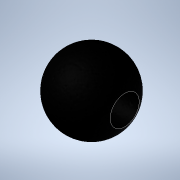
# Autodesk Inventor part: Ball
Saved by Autodesk Inventor 2022 (Build 260153000, 153)
## iProperties
Created: 2023-01-20
Part Number: Ball
Material: Generic
Document SubType Name: Modeling
Designer: ASUS
Density: 1 g/cm^3
Appearance: Fine Textured - Black
Author: ASUS
Autodesk Inventor part; units mm, degrees
ref_plane "XZ Plane" through (0, 0, 0) normal (0, 1, 0) x (-1, 0, 0)
ref_plane "XY Plane" through (0, 0, 0) normal (0, 0, 1) x (1, 0, 0)
sketch "Sketch1" plane through (0, 0, 0) normal (0, 1, 0) x (-1, 0, 0)
  arc A0 (25, 0) -> (-25, 0) centre (0, 0) ccw
  line L0 (25, 0) -> (-25, 0)
  dimension "d0" = 50
  constraints: 2 end point, 2 point on circle, 1 centre point, 1 coincident, 1 horizontal
  measures "d0" diameter of A0
revolve "Revolution1" add sketch "Sketch1" angle 360 about axis through (-25, 0, 0) along (1, 0, 0)
ref_plane "Work Plane1" through (22.5, 0, 0) normal (1, 0, 0) x (0, 1, 0)
sketch "Sketch2" plane through (22.5, 0, 0) normal (1, 0, 0) x (0, 1, 0)
  circle A0 centre (0, 0) radius 10
  dimension "d3" = 20
  constraints: 1 centre point, 1 coincident
  measures "d3" diameter of A0
extrude "Extrusion1" cut sketch "Sketch2" along normal blind 35 and the other way blind 35
sketch "Sketch3" plane through (0, 0, 0) normal (0, 0, 1) x (1, 0, 0)
  line L0 (-12.5, 10) -> (22.9129, 10) projected
  circle A0 centre (-2.5, 10) radius 2.25
  line L1 (22.9129, 10) -> (22.9129, -10) projected
  line L2 (-34.5826, 0) -> (32.4955, 0) projected
  point P0 (0, 0)
  point P1 (-0.25, 10)
  point P2 (-4.75, 10)
  dimension "d8" = 4.5
  dimension "d11" = 10
  constraints: 1 centre point, 1 point on line
  measures "d8" diameter of A0
  measures "d11" distance of L0.start A0.centre
revolve "Revolution2" add sketch "Sketch3" angle 360 about axis through (-10, 0, 0) along (1, 0, 0) picked at (-3.2282, 9.8205) contours L0 A0
body "Solid1"
